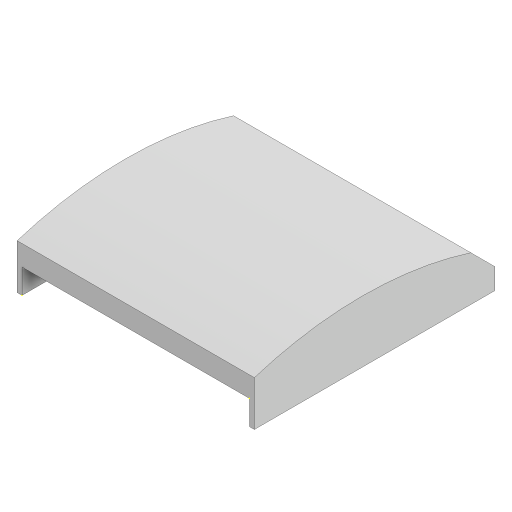
# Autodesk Inventor part: El capo
Saved by Autodesk Inventor 2024.3 (Build 283343000, 343)
## iProperties
Created: 2025-09-23
Part Number: El capo
Material: Generic
Document SubType Name: Modeling
Designer: danie
Density: 1 g/cm^3
Appearance: Default
Author: danie
Autodesk Inventor part; units mm, degrees
ref_plane "YZ Plane" through (0, 0, 0) normal (1, 0, 0) x (0, 1, 0)
ref_plane "XZ Plane" through (0, 0, 0) normal (0, 1, 0) x (-1, 0, 0)
ref_plane "XY Plane" through (0, 0, 0) normal (0, 0, 1) x (1, 0, 0)
sketch "Sketch1" plane through (0, 0, 0) normal (0, 1, 0) x (-1, 0, 0)
  line L0 (0, 0) -> (139.342, 0)
  line L1 (139.342, 0) -> (139.342, -147.342)
  line L2 (139.342, -147.342) -> (0, -147.342)
  line L3 (0, -147.342) -> (0, 0)
  line L4 (139.342, -147.342) -> (142.342, -147.342)
  line L5 (142.342, -147.342) -> (142.342, 0)
  line L6 (142.342, 0) -> (139.342, 0)
  line L7 (0, 0) -> (-3, 0)
  line L8 (-3, 0) -> (-3, -147.342)
  line L9 (-3, -147.342) -> (0, -147.342)
  dimension "d0" = 139.342
  dimension "d1" = 147.342
  dimension "d2" = 3
  dimension "d3" = 3
  constraints: 20 end point, 3 parallel, 2 collinear, 2 horizontal, 2 perpendicular, 2 point on line
  measures "d0" distance of L1.end L2.end
  measures "d1" distance of L0.end L1.end
  measures "d2" distance of L1.end L4.end
  measures "d3" distance of L0.start L7.end
extrude "Extrusion1" add sketch "Sketch1" along normal blind 15 contours L3 L9 L8 L7 | L6 L5 L4 L1
sketch "Sketch2" plane through (-139.342, 0, 0) normal (1, 0, 0) x (0, 0, -1)
  point P0 (0, 0)
sketch "Sketch3" plane through (0, 15, 0) normal (0, 1, 0) x (1, 0, 0)
  point P0 (0, 0)
sketch "Sketch4" plane through (0, 15, 0) normal (0, 1, 0) x (1, 0, 0)
  line L0 (-139.342, 147.342) -> (-142.342, 147.342) projected
  line L1 (0, 0) -> (3, 0) projected
  line L2 (-142.342, 147.342) -> (3, 147.342)
  line L3 (3, 147.342) -> (3, 0)
  line L4 (3, 0) -> (-142.342, 0)
  line L5 (-142.342, 0) -> (-142.342, 147.342)
  constraints: 8 end point, 2 parallel, 1 horizontal, 1 perpendicular
extrude "Extrusion2" add sketch "Sketch4" along normal blind 12.5
chamfer "Chamfer1" distance 14.75 angle 45 1 edges at (-69.671, 27.5, -147.342)
sketch "Sketch5" plane through (3, 0, 0) normal (1, 0, 0) x (0, 0, -1)
  line L0 (132.592, 27.5) -> (147.342, 12.75) projected
  arc A0 (132.592, 27.5) -> (0, 27.5) centre (66.296, -181.534) ccw
  line L1 (0, 27.5) -> (132.592, 27.5)
  point P0 (0, 0)
  constraints: 2 end point, 2 point on circle, 1 centre point, 1 point on line
extrude "Extrusion3" add sketch "Sketch5" against normal blind 145.342
sketch "Sketch6" plane through (-142.342, 0, -147.342) normal (-1, 0, 0) x (0, 0, 1)
  line L0 (147.342, 0) -> (147.342, 27.5) projected
  line L1 (147.342, 0) -> (147.342, 15)
  line L2 (0, 12.75) -> (14.75, 27.5) projected
  line L3 (147.342, 15) -> (0, 12.75)
  line L4 (0, 12.75) -> (1.9998, 12.7805)
  line L5 (1.9998, 12.7805) -> (15.7346, 26.5154)
  line L6 (147.342, 15) -> (145.3422, 14.9695)
  line L7 (145.3422, 14.9695) -> (145.1659, 26.5154)
  arc A0 (145.1659, 26.5154) -> (15.7346, 26.5154) centre (80.4503, -220.3584) ccw
  dimension "d13" = 15
  dimension "d14" = 2
  dimension "d15" = 2
  constraints: 12 end point, 4 point on line, 2 point on circle, 1 centre point, 1 perpendicular
  measures "d13" distance of L0.start L1.end
  measures "d14" distance of L2.start L4.end
  measures "d15" distance of L1.end L6.end
extrude "Extrusion4" cut sketch "Sketch6" against normal blind 142.342
sketch "Sketch7" plane through (-142.342, 0, -147.342) normal (-1, 0, 0) x (0, 0, 1)
  line L0 (1.9998, 12.7805) -> (145.3422, 14.9695) projected
  arc A0 (145.1659, 26.5154) -> (15.7346, 26.5154) centre (80.4503, -220.3584) ccw projected
  line L1 (1.9998, 12.7805) -> (15.7346, 26.5154)
  line L2 (145.1659, 26.5154) -> (145.3418, 15) projected
  line L3 (145.1659, 26.5154) -> (145.3418, 15)
  line L4 (145.3418, 15) -> (145.3418, 15)
  line L5 (1.9998, 12.7805) -> (145.3418, 15)
  arc A1 (145.1659, 26.5154) -> (15.7346, 26.5154) centre (80.4503, -220.3584) ccw
  point P0 (147.342, 0)
  constraints: 8 end point, 2 point on circle, 1 centre point, 1 collinear, 1 concentric
extrude "Extrusion5" add sketch "Sketch7" against normal blind 3.002
body "Solid1"
